Autodesk Fusion 360 part; units mm, degrees
(part 3 of 6)
  arc A18 (6.5769, 24.5337) -> (4.7192, 24.9577) centre (0, 0) ccw
  spline S7 degree 5 poles (4.7192, 24.9577) (4.7084, 24.9471) (4.6868, 24.9257) (4.6546, 24.8937) (4.6118, 24.8508) (4.5587, 24.797) (4.5059, 24.743) (4.4535, 24.6888) (4.4015, 24.6344) (4.3499, 24.5799) (4.2987, 24.5251) (4.2478, 24.4701) (4.1974, 24.415) (4.1473, 24.3596) (4.0977, 24.3041) (4.0484, 24.2484) (3.9995, 24.1925) (3.951, 24.1364) (3.903, 24.0801) (3.8553, 24.0236) (3.8081, 23.9669) (3.7613, 23.9101) (3.7149, 23.8531) (3.6689, 23.7958) (3.6234, 23.7385) (3.5783, 23.6809) (3.5336, 23.6231) (3.4894, 23.5652) (3.4456, 23.5071) (3.4023, 23.4488) (3.3594, 23.3903) (3.317, 23.3317) (3.275, 23.2729) (3.2335, 23.2139) (3.1925, 23.1547) (3.152, 23.0954) (3.1119, 23.0358) (3.0724, 22.9762) (3.0333, 22.9163) (2.9947, 22.8563) (2.9567, 22.7961) (2.9191, 22.7357) (2.8821, 22.6752) (2.8457, 22.6145) (2.8097, 22.5536) (2.7744, 22.4926) (2.7395, 22.4314) (2.7052, 22.37) (2.6715, 22.3085) (2.6383, 22.2468) (2.6058, 22.1849) (2.5738, 22.1229) (2.5426, 22.0607) (2.512, 21.9983) (2.4821, 21.9358) (2.4528, 21.873) (2.4242, 21.8102) (2.3961, 21.7472) (2.3686, 21.684) (2.3419, 21.6207) (2.316, 21.5572) (2.2911, 21.4935) (2.2673, 21.4296) (2.2446, 21.3655) (2.2228, 21.3011) (2.2018, 21.2367) (2.1812, 21.1721) (2.1613, 21.1075) (2.142, 21.0427) (2.1241, 20.9778) (2.1085, 20.9125) (2.0984, 20.8598) (2.0926, 20.82) (2.0895, 20.7934) (2.0882, 20.78) knots -1 -1 -1 -1 -1 -1 -0.98571429 -0.97142857 -0.95714286 -0.94285714 -0.92857143 -0.91428571 -0.9 -0.88571429 -0.87142857 -0.85714286 -0.84285714 -0.82857143 -0.81428571 -0.8 -0.78571429 -0.77142857 -0.75714286 -0.74285714 -0.72857143 -0.71428571 -0.7 -0.68571429 -0.67142857 -0.65714286 -0.64285714 -0.62857143 -0.61428571 -0.6 -0.58571429 -0.57142857 -0.55714286 -0.54285714 -0.52857143 -0.51428571 -0.5 -0.48571429 -0.47142857 -0.45714286 -0.44285714 -0.42857143 -0.41428571 -0.4 -0.38571429 -0.37142857 -0.35714286 -0.34285714 -0.32857143 -0.31428571 -0.3 -0.28571429 -0.27142857 -0.25714286 -0.24285714 -0.22857143 -0.21428571 -0.2 -0.18571429 -0.17142857 -0.15714286 -0.14285714 -0.12857143 -0.11428571 -0.1 -0.08571429 -0.07142857 -0.05714286 -0.04285714 -0.02857143 -0.01428571 0 0 0 0 0 0
  line L7 (2.0882, 20.78) -> (1.988, 19.788)
  arc A19 (0.376, 18.3604) -> (1.988, 19.788) centre (0.4085, 19.9475) ccw
  arc A20 (0.376, 18.3604) -> (-0.376, 18.3604) centre (0, 0) ccw
  arc A21 (-1.988, 19.788) -> (-0.376, 18.3604) centre (-0.4085, 19.9475) ccw
  line L8 (-1.988, 19.788) -> (-2.0882, 20.78)
  spline S8 degree 5 poles (-2.0882, 20.78) (-2.0895, 20.7934) (-2.0926, 20.82) (-2.0984, 20.8598) (-2.1085, 20.9125) (-2.1241, 20.9778) (-2.142, 21.0427) (-2.1613, 21.1075) (-2.1812, 21.1721) (-2.2018, 21.2367) (-2.2228, 21.3011) (-2.2446, 21.3655) (-2.2673, 21.4296) (-2.2911, 21.4935) (-2.316, 21.5572) (-2.3419, 21.6207) (-2.3686, 21.684) (-2.3961, 21.7472) (-2.4242, 21.8102) (-2.4528, 21.873) (-2.4821, 21.9358) (-2.512, 21.9983) (-2.5426, 22.0607) (-2.5738, 22.1229) (-2.6058, 22.1849) (-2.6383, 22.2468) (-2.6715, 22.3085) (-2.7052, 22.37) (-2.7395, 22.4314) (-2.7744, 22.4926) (-2.8097, 22.5536) (-2.8457, 22.6145) (-2.8821, 22.6752) (-2.9191, 22.7357) (-2.9567, 22.7961) (-2.9947, 22.8563) (-3.0333, 22.9163) (-3.0724, 22.9762) (-3.1119, 23.0358) (-3.152, 23.0954) (-3.1925, 23.1547) (-3.2335, 23.2139) (-3.275, 23.2729) (-3.317, 23.3317) (-3.3594, 23.3903) (-3.4023, 23.4488) (-3.4456, 23.5071) (-3.4894, 23.5652) (-3.5336, 23.6231) (-3.5783, 23.6809) (-3.6234, 23.7385) (-3.6689, 23.7958) (-3.7149, 23.8531) (-3.7613, 23.9101) (-3.8081, 23.9669) (-3.8553, 24.0236) (-3.903, 24.0801) (-3.951, 24.1364) (-3.9995, 24.1925) (-4.0484, 24.2484) (-4.0977, 24.3041) (-4.1473, 24.3596) (-4.1974, 24.415) (-4.2478, 24.4701) (-4.2987, 24.5251) (-4.3499, 24.5799) (-4.4015, 24.6344) (-4.4535, 24.6888) (-4.5059, 24.743) (-4.5587, 24.797) (-4.6118, 24.8508) (-4.6546, 24.8937) (-4.6868, 24.9257) (-4.7084, 24.9471) (-4.7192, 24.9577) knots 0 0 0 0 0 0 0.01428571 0.02857143 0.04285714 0.05714286 0.07142857 0.08571429 0.1 0.11428571 0.12857143 0.14285714 0.15714286 0.17142857 0.18571429 0.2 0.21428571 0.22857143 0.24285714 0.25714286 0.27142857 0.28571429 0.3 0.31428571 0.32857143 0.34285714 0.35714286 0.37142857 0.38571429 0.4 0.41428571 0.42857143 0.44285714 0.45714286 0.47142857 0.48571429 0.5 0.51428571 0.52857143 0.54285714 0.55714286 0.57142857 0.58571429 0.6 0.61428571 0.62857143 0.64285714 0.65714286 0.67142857 0.68571429 0.7 0.71428571 0.72857143 0.74285714 0.75714286 0.77142857 0.78571429 0.8 0.81428571 0.82857143 0.84285714 0.85714286 0.87142857 0.88571429 0.9 0.91428571 0.92857143 0.94285714 0.95714286 0.97142857 0.98571429 1 1 1 1 1 1
  arc A22 (-4.7192, 24.9577) -> (-6.5769, 24.5337) centre (0, 0) ccw
  spline S9 degree 5 poles (-6.5769, 24.5337) (-6.582, 24.5195) (-6.5922, 24.4909) (-6.6073, 24.448) (-6.6273, 24.3908) (-6.6518, 24.3193) (-6.6759, 24.2477) (-6.6996, 24.1762) (-6.7228, 24.1046) (-6.7457, 24.0331) (-6.768, 23.9615) (-6.79, 23.8899) (-6.8115, 23.8183) (-6.8326, 23.7467) (-6.8533, 23.6751) (-6.8735, 23.6036) (-6.8933, 23.532) (-6.9126, 23.4604) (-6.9315, 23.3888) (-6.9499, 23.3173) (-6.9679, 23.2457) (-6.9854, 23.1742) (-7.0024, 23.1027) (-7.019, 23.0312) (-7.0352, 22.9597) (-7.0508, 22.8883) (-7.066, 22.8169) (-7.0807, 22.7455) (-7.095, 22.6741) (-7.1087, 22.6028) (-7.122, 22.5315) (-7.1348, 22.4603) (-7.147, 22.3891) (-7.1588, 22.3179) (-7.1701, 22.2468) (-7.1809, 22.1758) (-7.1911, 22.1048) (-7.2009, 22.0339) (-7.2101, 21.963) (-7.2188, 21.8922) (-7.227, 21.8214) (-7.2346, 21.7507) (-7.2417, 21.6801) (-7.2482, 21.6096) (-7.2542, 21.5392) (-7.2595, 21.4689) (-7.2644, 21.3986) (-7.2687, 21.3284) (-7.2724, 21.2583) (-7.2755, 21.1884) (-7.278, 21.1185) (-7.2798, 21.0488) (-7.281, 20.9792) (-7.2814, 20.9097) (-7.2813, 20.8404) (-7.2804, 20.7712) (-7.279, 20.7021) (-7.277, 20.6332) (-7.2743, 20.5644) (-7.2709, 20.4957) (-7.2667, 20.4273) (-7.2615, 20.3591) (-7.2552, 20.2911) (-7.2478, 20.2235) (-7.2395, 20.1561) (-7.2305, 20.0889) (-7.221, 20.0218) (-7.211, 19.9549) (-7.2002, 19.8882) (-7.1881, 19.8219) (-7.1739, 19.7563) (-7.1601, 19.7045) (-7.1481, 19.6661) (-7.1393, 19.6408) (-7.1347, 19.6282) knots -1 -1 -1 -1 -1 -1 -0.98571429 -0.97142857 -0.95714286 -0.94285714 -0.92857143 -0.91428571 -0.9 -0.88571429 -0.87142857 -0.85714286 -0.84285714 -0.82857143 -0.81428571 -0.8 -0.78571429 -0.77142857 -0.75714286 -0.74285714 -0.72857143 -0.71428571 -0.7 -0.68571429 -0.67142857 -0.65714286 -0.64285714 -0.62857143 -0.61428571 -0.6 -0.58571429 -0.57142857 -0.55714286 -0.54285714 -0.52857143 -0.51428571 -0.5 -0.48571429 -0.47142857 -0.45714286 -0.44285714 -0.42857143 -0.41428571 -0.4 -0.38571429 -0.37142857 -0.35714286 -0.34285714 -0.32857143 -0.31428571 -0.3 -0.28571429 -0.27142857 -0.25714286 -0.24285714 -0.22857143 -0.21428571 -0.2 -0.18571429 -0.17142857 -0.15714286 -0.14285714 -0.12857143 -0.11428571 -0.1 -0.08571429 -0.07142857 -0.05714286 -0.04285714 -0.02857143 -0.01428571 0 0 0 0 0 0
  line L9 (-7.1347, 19.6282) -> (-6.7946, 18.6909)
  arc A23 (-7.6275, 16.7053) -> (-6.7946, 18.6909) centre (-8.2868, 18.1493) ccw
  arc A24 (-7.6275, 16.7053) -> (-8.305, 16.379) centre (0, 0) ccw
  arc A25 (-10.3768, 16.9658) -> (-8.305, 16.379) centre (-9.023, 17.7948) ccw
  line L10 (-10.3768, 16.9658) -> (-10.8975, 17.8161)
  spline S10 degree 5 poles (-10.8975, 17.8161) (-10.9045, 17.8276) (-10.9188, 17.8502) (-10.9414, 17.8836) (-10.9733, 17.9266) (-11.0157, 17.9787) (-11.06, 18.0295) (-11.1054, 18.0794) (-11.1515, 18.129) (-11.198, 18.1783) (-11.2449, 18.2272) (-11.2924, 18.2757) (-11.3407, 18.3237) (-11.3899, 18.3709) (-11.44, 18.4175) (-11.4908, 18.4635) (-11.5424, 18.5089) (-11.5946, 18.5539) (-11.6472, 18.5985) (-11.7003, 18.6427) (-11.7539, 18.6865) (-11.808, 18.7299) (-11.8626, 18.7728) (-11.9177, 18.8153) (-11.9734, 18.8573) (-12.0296, 18.8989) (-12.0862, 18.9401) (-12.1433, 18.9809) (-12.2008, 19.0213) (-12.2588, 19.0614) (-12.3171, 19.101) (-12.3759, 19.1403) (-12.4351, 19.1791) (-12.4947, 19.2176) (-12.5547, 19.2557) (-12.6151, 19.2934) (-12.6759, 19.3308) (-12.7371, 19.3678) (-12.7986, 19.4044) (-12.8605, 19.4406) (-12.9228, 19.4765) (-12.9854, 19.512) (-13.0484, 19.5472) (-13.1117, 19.5819) (-13.1754, 19.6164) (-13.2394, 19.6504) (-13.3037, 19.6842) (-13.3684, 19.7175) (-13.4334, 19.7505) (-13.4987, 19.7832) (-13.5643, 19.8155) (-13.6302, 19.8474) (-13.6965, 19.879) (-13.763, 19.9103) (-13.8298, 19.9412) (-13.897, 19.9717) (-13.9644, 20.0019) (-14.0321, 20.0318) (-14.1001, 20.0613) (-14.1684, 20.0905) (-14.237, 20.1193) (-14.3059, 20.1478) (-14.375, 20.176) (-14.4444, 20.2038) (-14.514, 20.2312) (-14.584, 20.2583) (-14.6541, 20.2851) (-14.7246, 20.3115) (-14.7953, 20.3376) (-14.8662, 20.3634) (-14.9374, 20.3888) (-14.9946, 20.4089) (-15.0376, 20.4238) (-15.0663, 20.4336) (-15.0806, 20.4385) knots 0 0 0 0 0 0 0.01428571 0.02857143 0.04285714 0.05714286 0.07142857 0.08571429 0.1 0.11428571 0.12857143 0.14285714 0.15714286 0.17142857 0.18571429 0.2 0.21428571 0.22857143 0.24285714 0.25714286 0.27142857 0.28571429 0.3 0.31428571 0.32857143 0.34285714 0.35714286 0.37142857 0.38571429 0.4 0.41428571 0.42857143 0.44285714 0.45714286 0.47142857 0.48571429 0.5 0.51428571 0.52857143 0.54285714 0.55714286 0.57142857 0.58571429 0.6 0.61428571 0.62857143 0.64285714 0.65714286 0.67142857 0.68571429 0.7 0.71428571 0.72857143 0.74285714 0.75714286 0.77142857 0.78571429 0.8 0.81428571 0.82857143 0.84285714 0.85714286 0.87142857 0.88571429 0.9 0.91428571 0.92857143 0.94285714 0.95714286 0.97142857 0.98571429 1 1 1 1 1 1
  arc A26 (-15.0806, 20.4385) -> (-16.5703, 19.2505) centre (0, 0) ccw
  spline S11 degree 5 poles (-16.5703, 19.2505) (-16.5688, 19.2354) (-16.5655, 19.2053) (-16.5606, 19.16) (-16.5537, 19.0999) (-16.5448, 19.0248) (-16.5355, 18.9499) (-16.5258, 18.8752) (-16.5157, 18.8006) (-16.5052, 18.7262) (-16.4943, 18.652) (-16.483, 18.578) (-16.4714, 18.5041) (-16.4593, 18.4305) (-16.4469, 18.357) (-16.434, 18.2838) (-16.4208, 18.2107) (-16.4071, 18.1378) (-16.3931, 18.0652) (-16.3786, 17.9927) (-16.3638, 17.9204) (-16.3485, 17.8484) (-16.3329, 17.7766) (-16.3168, 17.705) (-16.3003, 17.6336) (-16.2834, 17.5624) (-16.2661, 17.4915) (-16.2484, 17.4208) (-16.2303, 17.3503) (-16.2117, 17.2801) (-16.1927, 17.2101) (-16.1733, 17.1404) (-16.1535, 17.0709) (-16.1333, 17.0017) (-16.1126, 16.9327) (-16.0914, 16.864) (-16.0699, 16.7956) (-16.0479, 16.7275) (-16.0255, 16.6596) (-16.0026, 16.592) (-15.9792, 16.5247) (-15.9555, 16.4578) (-15.9312, 16.3911) (-15.9065, 16.3247) (-15.8813, 16.2587) (-15.8556, 16.193) (-15.8295, 16.1276) (-15.8029, 16.0625) (-15.7758, 15.9977) (-15.7483, 15.9334) (-15.7202, 15.8693) (-15.6916, 15.8057) (-15.6624, 15.7425) (-15.6327, 15.6797) (-15.6025, 15.6173) (-15.5717, 15.5553) (-15.5404, 15.4937) (-15.5087, 15.4325) (-15.4765, 15.3716) (-15.4436, 15.3113) (-15.4101, 15.2514) (-15.3758, 15.1922) (-15.3407, 15.1338) (-15.3047, 15.076) (-15.268, 15.0189) (-15.2307, 14.9622) (-15.193, 14.906) (-15.155, 14.85) (-15.1163, 14.7946) (-15.0767, 14.7401) (-15.0354, 14.6872) (-15.0005, 14.6465) (-14.973, 14.6171) (-14.9541, 14.5981) (-14.9445, 14.5887) knots -1 -1 -1 -1 -1 -1 -0.98571429 -0.97142857 -0.95714286 -0.94285714 -0.92857143 -0.91428571 -0.9 -0.88571429 -0.87142857 -0.85714286 -0.84285714 -0.82857143 -0.81428571 -0.8 -0.78571429 -0.77142857 -0.75714286 -0.74285714 -0.72857143 -0.71428571 -0.7 -0.68571429 -0.67142857 -0.65714286 -0.64285714 -0.62857143 -0.61428571 -0.6 -0.58571429 -0.57142857 -0.55714286 -0.54285714 -0.52857143 -0.51428571 -0.5 -0.48571429 -0.47142857 -0.45714286 -0.44285714 -0.42857143 -0.41428571 -0.4 -0.38571429 -0.37142857 -0.35714286 -0.34285714 -0.32857143 -0.31428571 -0.3 -0.28571429 -0.27142857 -0.25714286 -0.24285714 -0.22857143 -0.21428571 -0.2 -0.18571429 -0.17142857 -0.15714286 -0.14285714 -0.12857143 -0.11428571 -0.1 -0.08571429 -0.07142857 -0.05714286 -0.04285714 -0.02857143 -0.01428571 0 0 0 0 0 0
  line L11 (-14.9445, 14.5887) -> (-14.2314, 13.8919)
  arc A27 (-14.1203, 11.7415) -> (-14.2314, 13.8919) centre (-15.3409, 12.7565) ccw
  arc A28 (-14.1203, 11.7415) -> (-14.5891, 11.1535) centre (0, 0) ccw
  arc A29 (-16.7104, 10.7834) -> (-14.5891, 11.1535) centre (-15.8503, 12.1177) ccw
  line L12 (-16.7104, 10.7834) -> (-17.5484, 11.3235)
  spline S12 degree 5 poles (-17.5484, 11.3235) (-17.5597, 11.3308) (-17.5825, 11.345) (-17.6172, 11.3652) (-17.6646, 11.3902) (-17.7255, 11.4187) (-17.7874, 11.4452) (-17.85, 11.4706) (-17.913, 11.4952) (-17.9763, 11.5194) (-18.0398, 11.5432) (-18.1037, 11.5663) (-18.168, 11.5885) (-18.2328, 11.6097) (-18.2981, 11.63) (-18.3639, 11.6493) (-18.4301, 11.6679) (-18.4966, 11.6858) (-18.5633, 11.7031) (-18.6304, 11.7199) (-18.6976, 11.7361) (-18.7652, 11.7517) (-18.833, 11.7667) (-18.9011, 11.7811) (-18.9695, 11.7948) (-19.0382, 11.8079) (-19.1071, 11.8205) (-19.1762, 11.8324) (-19.2456, 11.8439) (-19.3152, 11.8548) (-19.385, 11.8652) (-19.455, 11.8751) (-19.5252, 11.8844) (-19.5956, 11.8932) (-19.6662, 11.9015) (-19.7369, 11.9093) (-19.8079, 11.9166) (-19.8791, 11.9233) (-19.9504, 11.9296) (-20.0219, 11.9354) (-20.0936, 11.9407) (-20.1654, 11.9455) (-20.2374, 11.9499) (-20.3095, 11.9538) (-20.3818, 11.9572) (-20.4543, 11.9601) (-20.5269, 11.9625) (-20.5996, 11.9645) (-20.6725, 11.9661) (-20.7455, 11.9672) (-20.8186, 11.9678) (-20.8919, 11.968) (-20.9653, 11.9677) (-21.0388, 11.967) (-21.1124, 11.9658) (-21.1862, 11.9642) (-21.26, 11.9622) (-21.334, 11.9597) (-21.4081, 11.9568) (-21.4823, 11.9535) (-21.5566, 11.9497) (-21.6309, 11.9455) (-21.7054, 11.9408) (-21.78, 11.9358) (-21.8547, 11.9303) (-21.9295, 11.9244) (-22.0043, 11.9181) (-22.0792, 11.9113) (-22.1543, 11.9041) (-22.2294, 11.8966) (-22.3045, 11.8886) (-22.3647, 11.8818) (-22.4099, 11.8766) (-22.4401, 11.8731) (-22.4551, 11.8712) knots 0 0 0 0 0 0 0.01428571 0.02857143 0.04285714 0.05714286 0.07142857 0.08571429 0.1 0.11428571 0.12857143 0.14285714 0.15714286 0.17142857 0.18571429 0.2 0.21428571 0.22857143 0.24285714 0.25714286 0.27142857 0.28571429 0.3 0.31428571 0.32857143 0.34285714 0.35714286 0.37142857 0.38571429 0.4 0.41428571 0.42857143 0.44285714 0.45714286 0.47142857 0.48571429 0.5 0.51428571 0.52857143 0.54285714 0.55714286 0.57142857 0.58571429 0.6 0.61428571 0.62857143 0.64285714 0.65714286 0.67142857 0.68571429 0.7 0.71428571 0.72857143 0.74285714 0.75714286 0.77142857 0.78571429 0.8 0.81428571 0.82857143 0.84285714 0.85714286 0.87142857 0.88571429 0.9 0.91428571 0.92857143 0.94285714 0.95714286 0.97142857 0.98571429 1 1 1 1 1 1
  arc A30 (-22.4551, 11.8712) -> (-23.2819, 10.1545) centre (0, 0) ccw
  spline S13 degree 5 poles (-23.2819, 10.1545) (-23.2739, 10.1416) (-23.2579, 10.1158) (-23.2338, 10.0772) (-23.2015, 10.026) (-23.1609, 9.9622) (-23.12, 9.8988) (-23.0788, 9.8357) (-23.0374, 9.7729) (-22.9956, 9.7104) (-22.9537, 9.6483) (-22.9114, 9.5865) (-22.8688, 9.525) (-22.826, 9.4639) (-22.7829, 9.4031) (-22.7396, 9.3426) (-22.6959, 9.2826) (-22.652, 9.2228) (-22.6078, 9.1634) (-22.5634, 9.1044) (-22.5186, 9.0458) (-22.4736, 8.9875) (-22.4284, 8.9296) (-22.3828, 8.872) (-22.337, 8.8148) (-22.2909, 8.7581) (-22.2445, 8.7017) (-22.1979, 8.6456) (-22.151, 8.59) (-22.1038, 8.5348) (-22.0563, 8.48) (-22.0086, 8.4256) (-21.9606, 8.3716) (-21.9123, 8.318) (-21.8638, 8.2649) (-21.8149, 8.2122) (-21.7658, 8.1599) (-21.7164, 8.108) (-21.6668, 8.0566) (-21.6168, 8.0056) (-21.5666, 7.9551) (-21.5161, 7.9051) (-21.4653, 7.8556) (-21.4143, 7.8065) (-21.3629, 7.7579) (-21.3113, 7.7099) (-21.2594, 7.6623) (-21.2072, 7.6152) (-21.1547, 7.5686) (-21.1019, 7.5225) (-21.0489, 7.477) (-20.9955, 7.4321) (-20.9418, 7.3878) (-20.8878, 7.3441) (-20.8335, 7.3011) (-20.7788, 7.2586) (-20.7239, 7.2166) (-20.6688, 7.1752) (-20.6133, 7.1344) (-20.5575, 7.0942) (-20.5014, 7.0549) (-20.4448, 7.0164) (-20.3878, 6.979) (-20.3303, 6.9426) (-20.2724, 6.907) (-20.2143, 6.8722) (-20.1559, 6.8378) (-20.0973, 6.8039) (-20.0385, 6.7707) (-19.9791, 6.7389) (-19.919, 6.7091) (-19.8699, 6.6876) (-19.8324, 6.673) (-19.8071, 6.6641) (-19.7944, 6.6598) knots -1 -1 -1 -1 -1 -1 -0.98571429 -0.97142857 -0.95714286 -0.94285714 -0.92857143 -0.91428571 -0.9 -0.88571429 -0.87142857 -0.85714286 -0.84285714 -0.82857143 -0.81428571 -0.8 -0.78571429 -0.77142857 -0.75714286 -0.74285714 -0.72857143 -0.71428571 -0.7 -0.68571429 -0.67142857 -0.65714286 -0.64285714 -0.62857143 -0.61428571 -0.6 -0.58571429 -0.57142857 -0.55714286 -0.54285714 -0.52857143 -0.51428571 -0.5 -0.48571429 -0.47142857 -0.45714286 -0.44285714 -0.42857143 -0.41428571 -0.4 -0.38571429 -0.37142857 -0.35714286 -0.34285714 -0.32857143 -0.31428571 -0.3 -0.28571429 -0.27142857 -0.25714286 -0.24285714 -0.22857143 -0.21428571 -0.2 -0.18571429 -0.17142857 -0.15714286 -0.14285714 -0.12857143 -0.11428571 -0.1 -0.08571429 -0.07142857 -0.05714286 -0.04285714 -0.02857143 -0.01428571 0 0 0 0 0 0
  line L13 (-19.7944, 6.6598) -> (-18.8495, 6.3414)
  arc A31 (-17.8163, 4.4521) -> (-18.8495, 6.3414) centre (-19.3565, 4.837) ccw
  arc A32 (-17.8163, 4.4521) -> (-17.9837, 3.719) centre (0, 0) ccw
  arc A33 (-19.7343, 2.4651) -> (-17.9837, 3.719) centre (-19.5383, 4.0405) ccw
  line L14 (-19.7343, 2.4651) -> (-20.7237, 2.5882)
  spline S14 degree 5 poles (-20.7237, 2.5882) (-20.737, 2.5898) (-20.7637, 2.5928) (-20.8037, 2.5959) (-20.8573, 2.5978) (-20.9245, 2.5971) (-20.9918, 2.5941) (-21.0592, 2.5898) (-21.1266, 2.5847) (-21.1941, 2.5791) (-21.2617, 2.5729) (-21.3292, 2.566) (-21.3968, 2.5581) (-21.4645, 2.5491) (-21.5321, 2.539) (-21.5998, 2.5279) (-21.6674, 2.5159) (-21.7351, 2.5032) (-21.8028, 2.4898) (-21.8705, 2.4759) (-21.9381, 2.4613) (-22.0057, 2.446) (-22.0734, 2.4301) (-22.141, 2.4135) (-22.2085, 2.3962) (-22.2761, 2.3782) (-22.3436, 2.3596) (-22.4111, 2.3404) (-22.4786, 2.3206) (-22.546, 2.3003) (-22.6134, 2.2794) (-22.6807, 2.2579) (-22.748, 2.2358) (-22.8153, 2.2132) (-22.8825, 2.1901) (-22.9496, 2.1664) (-23.0167, 2.1421) (-23.0838, 2.1173) (-23.1508, 2.092) (-23.2177, 2.0662) (-23.2846, 2.0399) (-23.3514, 2.0131) (-23.4181, 1.9858) (-23.4848, 1.958) (-23.5514, 1.9297) (-23.618, 1.9009) (-23.6844, 1.8716) (-23.7508, 1.8418) (-23.8171, 1.8116) (-23.8834, 1.7809) (-23.9496, 1.7498) (-24.0156, 1.7181) (-24.0817, 1.686) (-24.1476, 1.6535) (-24.2134, 1.6205) (-24.2792, 1.5871) (-24.3448, 1.5532) (-24.4104, 1.5189) (-24.4759, 1.4841) (-24.5413, 1.4489) (-24.6066, 1.4133) (-24.6718, 1.3772) (-24.7369, 1.3407) (-24.8019, 1.3038) (-24.8668, 1.2664) (-24.9316, 1.2287) (-24.9962, 1.1905) (-25.0608, 1.1519) (-25.1253, 1.1129) (-25.1897, 1.0735) (-25.2539, 1.0337) (-25.3053, 1.0015) (-25.3437, 0.9772) (-25.3693, 0.9609) (-25.3821, 0.9527) knots 0 0 0 0 0 0 0.01428571 0.02857143 0.04285714 0.05714286 0.07142857 0.08571429 0.1 0.11428571 0.12857143 0.14285714 0.15714286 0.17142857 0.18571429 0.2 0.21428571 0.22857143 0.24285714 0.25714286 0.27142857 0.28571429 0.3 0.31428571 0.32857143 0.34285714 0.35714286 0.37142857 0.38571429 0.4 0.41428571 0.42857143 0.44285714 0.45714286 0.47142857 0.48571429 0.5 0.51428571 0.52857143 0.54285714 0.55714286 0.57142857 0.58571429 0.6 0.61428571 0.62857143 0.64285714 0.65714286 0.67142857 0.68571429 0.7 0.71428571 0.72857143 0.74285714 0.75714286 0.77142857 0.78571429 0.8 0.81428571 0.82857143 0.84285714 0.85714286 0.87142857 0.88571429 0.9 0.91428571 0.92857143 0.94285714 0.95714286 0.97142857 0.98571429 1 1 1 1 1 1
  arc A34 (-25.3821, 0.9527) -> (-25.3821, -0.9527) centre (0, 0) ccw
  spline S15 degree 5 poles (-25.3821, -0.9527) (-25.3693, -0.9609) (-25.3437, -0.9772) (-25.3053, -1.0015) (-25.2539, -1.0337) (-25.1897, -1.0735) (-25.1253, -1.1129) (-25.0608, -1.1519) (-24.9962, -1.1905) (-24.9316, -1.2287) (-24.8668, -1.2664) (-24.8019, -1.3038) (-24.7369, -1.3407) (-24.6718, -1.3772) (-24.6066, -1.4133) (-24.5413, -1.4489) (-24.4759, -1.4841) (-24.4104, -1.5189) (-24.3448, -1.5532) (-24.2792, -1.5871) (-24.2134, -1.6205) (-24.1476, -1.6535) (-24.0817, -1.686) (-24.0156, -1.7181) (-23.9496, -1.7498) (-23.8834, -1.7809) (-23.8171, -1.8116) (-23.7508, -1.8418) (-23.6844, -1.8716) (-23.618, -1.9009) (-23.5514, -1.9297) (-23.4848, -1.958) (-23.4181, -1.9858) (-23.3514, -2.0131) (-23.2846, -2.0399) (-23.2177, -2.0662) (-23.1508, -2.092) (-23.0838, -2.1173) (-23.0167, -2.1421) (-22.9496, -2.1664) (-22.8825, -2.1901) (-22.8153, -2.2132) (-22.748, -2.2358) (-22.6807, -2.2579) (-22.6134, -2.2794) (-22.546, -2.3003) (-22.4786, -2.3206) (-22.4111, -2.3404) (-22.3436, -2.3596) (-22.2761, -2.3782) (-22.2085, -2.3962) (-22.141, -2.4135) (-22.0734, -2.4301) (-22.0057, -2.446) (-21.9381, -2.4613) (-21.8705, -2.4759) (-21.8028, -2.4898) (-21.7351, -2.5032) (-21.6674, -2.5159) (-21.5998, -2.5279) (-21.5321, -2.539) (-21.4645, -2.5491) (-21.3968, -2.5581) (-21.3292, -2.566) (-21.2617, -2.5729) (-21.1941, -2.5791) (-21.1266, -2.5847) (-21.0592, -2.5898) (-20.9918, -2.5941) (-20.9245, -2.5971) (-20.8573, -2.5978) (-20.8037, -2.5959) (-20.7637, -2.5928) (-20.737, -2.5898) (-20.7237, -2.5882) knots -1 -1 -1 -1 -1 -1 -0.98571429 -0.97142857 -0.95714286 -0.94285714 -0.92857143 -0.91428571 -0.9 -0.88571429 -0.87142857 -0.85714286 -0.84285714 -0.82857143 -0.81428571 -0.8 -0.78571429 -0.77142857 -0.75714286 -0.74285714 -0.72857143 -0.71428571 -0.7 -0.68571429 -0.67142857 -0.65714286 -0.64285714 -0.62857143 -0.61428571 -0.6 -0.58571429 -0.57142857 -0.55714286 -0.54285714 -0.52857143 -0.51428571 -0.5 -0.48571429 -0.47142857 -0.45714286 -0.44285714 -0.42857143 -0.41428571 -0.4 -0.38571429 -0.37142857 -0.35714286 -0.34285714 -0.32857143 -0.31428571 -0.3 -0.28571429 -0.27142857 -0.25714286 -0.24285714 -0.22857143 -0.21428571 -0.2 -0.18571429 -0.17142857 -0.15714286 -0.14285714 -0.12857143 -0.11428571 -0.1 -0.08571429 -0.07142857 -0.05714286 -0.04285714 -0.02857143 -0.01428571 0 0 0 0 0 0
  line L15 (-20.7237, -2.5882) -> (-19.7343, -2.4651)
  arc A35 (-17.9837, -3.719) -> (-19.7343, -2.4651) centre (-19.5383, -4.0405) ccw
  arc A36 (-17.9837, -3.719) -> (-17.8163, -4.4521) centre (0, 0) ccw
  arc A37 (-18.8495, -6.3414) -> (-17.8163, -4.4521) centre (-19.3565, -4.837) ccw
  line L16 (-18.8495, -6.3414) -> (-19.7944, -6.6598)
  spline S16 degree 5 poles (-19.7944, -6.6598) (-19.8071, -6.6641) (-19.8324, -6.673) (-19.8699, -6.6876) (-19.919, -6.7091) (-19.9791, -6.7389) (-20.0385, -6.7707) (-20.0973, -6.8039) (-20.1559, -6.8378) (-20.2143, -6.8722) (-20.2724, -6.907) (-20.3303, -6.9426) (-20.3878, -6.979) (-20.4448, -7.0164) (-20.5014, -7.0549) (-20.5575, -7.0942) (-20.6133, -7.1344) (-20.6688, -7.1752) (-20.7239, -7.2166) (-20.7788, -7.2586) (-20.8335, -7.3011) (-20.8878, -7.3441) (-20.9418, -7.3878) (-20.9955, -7.4321) (-21.0489, -7.477) (-21.1019, -7.5225) (-21.1547, -7.5686) (-21.2072, -7.6152) (-21.2594, -7.6623) (-21.3113, -7.7099) (-21.3629, -7.7579) (-21.4143, -7.8065) (-21.4653, -7.8556) (-21.5161, -7.9051) (-21.5666, -7.9551) (-21.6168, -8.0056) (-21.6668, -8.0566) (-21.7164, -8.108) (-21.7658, -8.1599) (-21.8149, -8.2122) (-21.8638, -8.2649) (-21.9123, -8.318) (-21.9606, -8.3716) (-22.0086, -8.4256) (-22.0563, -8.48) (-22.1038, -8.5348) (-22.151, -8.59) (-22.1979, -8.6456) (-22.2445, -8.7017) (-22.2909, -8.7581) (-22.337, -8.8148) (-22.3828, -8.872) (-22.4284, -8.9296) (-22.4736, -8.9875) (-22.5186, -9.0458) (-22.5634, -9.1044) (-22.6078, -9.1634) (-22.652, -9.2228) (-22.6959, -9.2826) (-22.7396, -9.3426) (-22.7829, -9.4031) (-22.826, -9.4639) (-22.8688, -9.525) (-22.9114, -9.5865) (-22.9537, -9.6483) (-22.9956, -9.7104) (-23.0374, -9.7729) (-23.0788, -9.8357) (-23.12, -9.8988) (-23.1609, -9.9622) (-23.2015, -10.026) (-23.2338, -10.0772) (-23.2579, -10.1158) (-23.2739, -10.1416) (-23.2819, -10.1545) knots 0 0 0 0 0 0 0.01428571 0.02857143 0.04285714 0.05714286 0.07142857 0.08571429 0.1 0.11428571 0.12857143 0.14285714 0.15714286 0.17142857 0.18571429 0.2 0.21428571 0.22857143 0.24285714 0.25714286 0.27142857 0.28571429 0.3 0.31428571 0.32857143 0.34285714 0.35714286 0.37142857 0.38571429 0.4 0.41428571 0.42857143 0.44285714 0.45714286 0.47142857 0.48571429 0.5 0.51428571 0.52857143 0.54285714 0.55714286 0.57142857 0.58571429 0.6 0.61428571 0.62857143 0.64285714 0.65714286 0.67142857 0.68571429 0.7 0.71428571 0.72857143 0.74285714 0.75714286 0.77142857 0.78571429 0.8 0.81428571 0.82857143 0.84285714 0.85714286 0.87142857 0.88571429 0.9 0.91428571 0.92857143 0.94285714 0.95714286 0.97142857 0.98571429 1 1 1 1 1 1
  arc A38 (-23.2819, -10.1545) -> (-22.4551, -11.8712) centre (0, 0) ccw
  spline S17 degree 5 poles (-22.4551, -11.8712) (-22.4401, -11.8731) (-22.4099, -11.8766) (-22.3647, -11.8818) (-22.3045, -11.8886) (-22.2294, -11.8966) (-22.1543, -11.9041) (-22.0792, -11.9113) (-22.0043, -11.9181) (-21.9295, -11.9244) (-21.8547, -11.9303) (-21.78, -11.9358) (-21.7054, -11.9408) (-21.6309, -11.9455) (-21.5566, -11.9497) (-21.4823, -11.9535) (-21.4081, -11.9568) (-21.334, -11.9597) (-21.26, -11.9622) (-21.1862, -11.9642) (-21.1124, -11.9658) (-21.0388, -11.967) (-20.9653, -11.9677) (-20.8919, -11.968) (-20.8186, -11.9678) (-20.7455, -11.9672) (-20.6725, -11.9661) (-20.5996, -11.9645) (-20.5269, -11.9625) (-20.4543, -11.9601) (-20.3818, -11.9572) (-20.3095, -11.9538) (-20.2374, -11.9499) (-20.1654, -11.9455) (-20.0936, -11.9407) (-20.0219, -11.9354) (-19.9504, -11.9296) (-19.8791, -11.9233) (-19.8079, -11.9166) (-19.7369, -11.9093) (-19.6662, -11.9015) (-19.5956, -11.8932) (-19.5252, -11.8844) (-19.455, -11.8751) (-19.385, -11.8652) (-19.3152, -11.8548) (-19.2456, -11.8439) (-19.1762, -11.8324) (-19.1071, -11.8205) (-19.0382, -11.8079) (-18.9695, -11.7948) (-18.9011, -11.7811) (-18.833, -11.7667) (-18.7652, -11.7517) (-18.6976, -11.7361) (-18.6304, -11.7199) (-18.5633, -11.7031) (-18.4966, -11.6858) (-18.4301, -11.6679) (-18.3639, -11.6493) (-18.2981, -11.63) (-18.2328, -11.6097) (-18.168, -11.5885) (-18.1037, -11.5663) (-18.0398, -11.5432) (-17.9763, -11.5194) (-17.913, -11.4952) (-17.85, -11.4706) (-17.7874, -11.4452) (-17.7255, -11.4187) (-17.6646, -11.3902) (-17.6172, -11.3652) (-17.5825, -11.345) (-17.5597, -11.3308) (-17.5484, -11.3235) knots -1 -1 -1 -1 -1 -1 -0.98571429 -0.97142857 -0.95714286 -0.94285714 -0.92857143 -0.91428571 -0.9 -0.88571429 -0.87142857 -0.85714286 -0.84285714 -0.82857143 -0.81428571 -0.8 -0.78571429 -0.77142857 -0.75714286 -0.74285714 -0.72857143 -0.71428571 -0.7 -0.68571429 -0.67142857 -0.65714286 -0.64285714 -0.62857143 -0.61428571 -0.6 -0.58571429 -0.57142857 -0.55714286 -0.54285714 -0.52857143 -0.51428571 -0.5 -0.48571429 -0.47142857 -0.45714286 -0.44285714 -0.42857143 -0.41428571 -0.4 -0.38571429 -0.37142857 -0.35714286 -0.34285714 -0.32857143 -0.31428571 -0.3 -0.28571429 -0.27142857 -0.25714286 -0.24285714 -0.22857143 -0.21428571 -0.2 -0.18571429 -0.17142857 -0.15714286 -0.14285714 -0.12857143 -0.11428571 -0.1 -0.08571429 -0.07142857 -0.05714286 -0.04285714 -0.02857143 -0.01428571 0 0 0 0 0 0
  line L17 (-17.5484, -11.3235) -> (-16.7104, -10.7834)
  arc A39 (-14.5891, -11.1535) -> (-16.7104, -10.7834) centre (-15.8503, -12.1177) ccw
  arc A40 (-14.5891, -11.1535) -> (-14.1203, -11.7415) centre (0, 0) ccw
  arc A41 (-14.2314, -13.8919) -> (-14.1203, -11.7415) centre (-15.3409, -12.7565) ccw
  line L18 (-14.2314, -13.8919) -> (-14.9445, -14.5887)
  spline S18 degree 5 poles (-14.9445, -14.5887) (-14.9541, -14.5981) (-14.973, -14.6171) (-15.0005, -14.6465) (-15.0354, -14.6872) (-15.0767, -14.7401) (-15.1163, -14.7946) (-15.155, -14.85) (-15.193, -14.906) (-15.2307, -14.9622) (-15.268, -15.0189) (-15.3047, -15.076) (-15.3407, -15.1338) (-15.3758, -15.1922) (-15.4101, -15.2514) (-15.4436, -15.3113) (-15.4765, -15.3716) (-15.5087, -15.4325) (-15.5404, -15.4937) (-15.5717, -15.5553) (-15.6025, -15.6173) (-15.6327, -15.6797) (-15.6624, -15.7425) (-15.6916, -15.8057) (-15.7202, -15.8693) (-15.7483, -15.9334) (-15.7758, -15.9977) (-15.8029, -16.0625) (-15.8295, -16.1276) (-15.8556, -16.193) (-15.8813, -16.2587) (-15.9065, -16.3247) (-15.9312, -16.3911) (-15.9555, -16.4578) (-15.9792, -16.5247) (-16.0026, -16.592) (-16.0255, -16.6596) (-16.0479, -16.7275) (-16.0699, -16.7956) (-16.0914, -16.864) (-16.1126, -16.9327) (-16.1333, -17.0017) (-16.1535, -17.0709) (-16.1733, -17.1404) (-16.1927, -17.2101) (-16.2117, -17.2801) (-16.2303, -17.3503) (-16.2484, -17.4208) (-16.2661, -17.4915) (-16.2834, -17.5624) (-16.3003, -17.6336) (-16.3168, -17.705) (-16.3329, -17.7766) (-16.3485, -17.8484) (-16.3638, -17.9204) (-16.3786, -17.9927) (-16.3931, -18.0652) (-16.4071, -18.1378) (-16.4208, -18.2107) (-16.434, -18.2838) (-16.4469, -18.357) (-16.4593, -18.4305) (-16.4714, -18.5041) (-16.483, -18.578) (-16.4943, -18.652) (-16.5052, -18.7262) (-16.5157, -18.8006) (-16.5258, -18.8752) (-16.5355, -18.9499) (-16.5448, -19.0248) (-16.5537, -19.0999) (-16.5606, -19.16) (-16.5655, -19.2053) (-16.5688, -19.2354) (-16.5703, -19.2505) knots 0 0 0 0 0 0 0.01428571 0.02857143 0.04285714 0.05714286 0.07142857 0.08571429 0.1 0.11428571 0.12857143 0.14285714 0.15714286 0.17142857 0.18571429 0.2 0.21428571 0.22857143 0.24285714 0.25714286 0.27142857 0.28571429 0.3 0.31428571 0.32857143 0.34285714 0.35714286 0.37142857 0.38571429 0.4 0.41428571 0.42857143 0.44285714 0.45714286 0.47142857 0.48571429 0.5 0.51428571 0.52857143 0.54285714 0.55714286 0.57142857 0.58571429 0.6 0.61428571 0.62857143 0.64285714 0.65714286 0.67142857 0.68571429 0.7 0.71428571 0.72857143 0.74285714 0.75714286 0.77142857 0.78571429 0.8 0.81428571 0.82857143 0.84285714 0.85714286 0.87142857 0.88571429 0.9 0.91428571 0.92857143 0.94285714 0.95714286 0.97142857 0.98571429 1 1 1 1 1 1
  arc A42 (-16.5703, -19.2505) -> (-15.0806, -20.4385) centre (0, 0) ccw
  spline S19 degree 5 poles (-15.0806, -20.4385) (-15.0663, -20.4336) (-15.0376, -20.4238) (-14.9946, -20.4089) (-14.9374, -20.3888) (-14.8662, -20.3634) (-14.7953, -20.3376) (-14.7246, -20.3115) (-14.6541, -20.2851) (-14.584, -20.2583) (-14.514, -20.2312) (-14.4444, -20.2038) (-14.375, -20.176) (-14.3059, -20.1478) (-14.237, -20.1193) (-14.1684, -20.0905) (-14.1001, -20.0613) (-14.0321, -20.0318) (-13.9644, -20.0019) (-13.897, -19.9717) (-13.8298, -19.9412) (-13.763, -19.9103) (-13.6965, -19.879) (-13.6302, -19.8474) (-13.5643, -19.8155) (-13.4987, -19.7832) (-13.4334, -19.7505) (-13.3684, -19.7175) (-13.3037, -19.6842) (-13.2394, -19.6504) (-13.1754, -19.6164) (-13.1117, -19.5819) (-13.0484, -19.5472) (-12.9854, -19.512) (-12.9228, -19.4765) (-12.8605, -19.4406) (-12.7986, -19.4044) (-12.7371, -19.3678) (-12.6759, -19.3308) (-12.6151, -19.2934) (-12.5547, -19.2557) (-12.4947, -19.2176) (-12.4351, -19.1791) (-12.3759, -19.1403) (-12.3171, -19.101) (-12.2588, -19.0614) (-12.2008, -19.0213) (-12.1433, -18.9809) (-12.0862, -18.9401) (-12.0296, -18.8989) (-11.9734, -18.8573) (-11.9177, -18.8153) (-11.8626, -18.7728) (-11.808, -18.7299) (-11.7539, -18.6865) (-11.7003, -18.6427) (-11.6472, -18.5985) (-11.5946, -18.5539) (-11.5424, -18.5089) (-11.4908, -18.4635) (-11.44, -18.4175) (-11.3899, -18.3709) (-11.3407, -18.3237) (-11.2924, -18.2757) (-11.2449, -18.2272) (-11.198, -18.1783) (-11.1515, -18.129) (-11.1054, -18.0794) (-11.06, -18.0295) (-11.0157, -17.9787) (-10.9733, -17.9266) (-10.9414, -17.8836) (-10.9188, -17.8502) (-10.9045, -17.8276) (-10.8975, -17.8161) knots -1 -1 -1 -1 -1 -1 -0.98571429 -0.97142857 -0.95714286 -0.94285714 -0.92857143 -0.91428571 -0.9 -0.88571429 -0.87142857 -0.85714286 -0.84285714 -0.82857143 -0.81428571 -0.8 -0.78571429 -0.77142857 -0.75714286 -0.74285714 -0.72857143 -0.71428571 -0.7 -0.68571429 -0.67142857 -0.65714286 -0.64285714 -0.62857143 -0.61428571 -0.6 -0.58571429 -0.57142857 -0.55714286 -0.54285714 -0.52857143 -0.51428571 -0.5 -0.48571429 -0.47142857 -0.45714286 -0.44285714 -0.42857143 -0.41428571 -0.4 -0.38571429 -0.37142857 -0.35714286 -0.34285714 -0.32857143 -0.31428571 -0.3 -0.28571429 -0.27142857 -0.25714286 -0.24285714 -0.22857143 -0.21428571 -0.2 -0.18571429 -0.17142857 -0.15714286 -0.14285714 -0.12857143 -0.11428571 -0.1 -0.08571429 -0.07142857 -0.05714286 -0.04285714 -0.02857143 -0.01428571 0 0 0 0 0 0
  line L19 (-10.8975, -17.8161) -> (-10.3768, -16.9658)
  arc A43 (-8.305, -16.379) -> (-10.3768, -16.9658) centre (-9.023, -17.7948) ccw
  arc A44 (-8.305, -16.379) -> (-7.6275, -16.7053) centre (0, 0) ccw
  arc A45 (-6.7946, -18.6909) -> (-7.6275, -16.7053) centre (-8.2868, -18.1493) ccw
  line L20 (-6.7946, -18.6909) -> (-7.1347, -19.6282)
  spline S20 degree 5 poles (-7.1347, -19.6282) (-7.1393, -19.6408) (-7.1481, -19.6661) (-7.1601, -19.7045) (-7.1739, -19.7563) (-7.1881, -19.8219) (-7.2002, -19.8882) (-7.211, -19.9549) (-7.221, -20.0218) (-7.2305, -20.0889) (-7.2395, -20.1561) (-7.2478, -20.2235) (-7.2552, -20.2911) (-7.2615, -20.3591) (-7.2667, -20.4273) (-7.2709, -20.4957) (-7.2743, -20.5644) (-7.277, -20.6332) (-7.279, -20.7021) (-7.2804, -20.7712) (-7.2813, -20.8404) (-7.2814, -20.9097) (-7.281, -20.9792) (-7.2798, -21.0488) (-7.278, -21.1185) (-7.2755, -21.1884) (-7.2724, -21.2583) (-7.2687, -21.3284) (-7.2644, -21.3986) (-7.2595, -21.4689) (-7.2542, -21.5392) (-7.2482, -21.6096) (-7.2417, -21.6801) (-7.2346, -21.7507) (-7.227, -21.8214) (-7.2188, -21.8922) (-7.2101, -21.963) (-7.2009, -22.0339) (-7.1911, -22.1048) (-7.1809, -22.1758) (-7.1701, -22.2468) (-7.1588, -22.3179) (-7.147, -22.3891) (-7.1348, -22.4603) (-7.122, -22.5315) (-7.1087, -22.6028) (-7.095, -22.6741) (-7.0807, -22.7455) (-7.066, -22.8169) (-7.0508, -22.8883) (-7.0352, -22.9597) (-7.019, -23.0312) (-7.0024, -23.1027) (-6.9854, -23.1742) (-6.9679, -23.2457) (-6.9499, -23.3173) (-6.9315, -23.3888) (-6.9126, -23.4604) (-6.8933, -23.532) (-6.8735, -23.6036) (-6.8533, -23.6751) (-6.8326, -23.7467) (-6.8115, -23.8183) (-6.79, -23.8899) (-6.768, -23.9615) (-6.7457, -24.0331) (-6.7228, -24.1046) (-6.6996, -24.1762) (-6.6759, -24.2477) (-6.6518, -24.3193) (-6.6273, -24.3908) (-6.6073, -24.448) (-6.5922, -24.4909) (-6.582, -24.5195) (-6.5769, -24.5337) knots 0 0 0 0 0 0 0.01428571 0.02857143 0.04285714 0.05714286 0.07142857 0.08571429 0.1 0.11428571 0.12857143 0.14285714 0.15714286 0.17142857 0.18571429 0.2 0.21428571 0.22857143 0.24285714 0.25714286 0.27142857 0.28571429 0.3 0.31428571 0.32857143 0.34285714 0.35714286 0.37142857 0.38571429 0.4 0.41428571 0.42857143 0.44285714 0.45714286 0.47142857 0.48571429 0.5 0.51428571 0.52857143 0.54285714 0.55714286 0.57142857 0.58571429 0.6 0.61428571 0.62857143 0.64285714 0.65714286 0.67142857 0.68571429 0.7 0.71428571 0.72857143 0.74285714 0.75714286 0.77142857 0.78571429 0.8 0.81428571 0.82857143 0.84285714 0.85714286 0.87142857 0.88571429 0.9 0.91428571 0.92857143 0.94285714 0.95714286 0.97142857 0.98571429 1 1 1 1 1 1
  arc A46 (-6.5769, -24.5337) -> (-4.7192, -24.9577) centre (0, 0) ccw
  spline S21 degree 5 poles (-4.7192, -24.9577) (-4.7084, -24.9471) (-4.6868, -24.9257) (-4.6546, -24.8937) (-4.6118, -24.8508) (-4.5587, -24.797) (-4.5059, -24.743) (-4.4535, -24.6888) (-4.4015, -24.6344) (-4.3499, -24.5799) (-4.2987, -24.5251) (-4.2478, -24.4701) (-4.1974, -24.415) (-4.1473, -24.3596) (-4.0977, -24.3041) (-4.0484, -24.2484) (-3.9995, -24.1925) (-3.951, -24.1364) (-3.903, -24.0801) (-3.8553, -24.0236) (-3.8081, -23.9669) (-3.7613, -23.9101) (-3.7149, -23.8531) (-3.6689, -23.7958) (-3.6234, -23.7385) (-3.5783, -23.6809) (-3.5336, -23.6231) (-3.4894, -23.5652) (-3.4456, -23.5071) (-3.4023, -23.4488) (-3.3594, -23.3903) (-3.317, -23.3317) (-3.275, -23.2729) (-3.2335, -23.2139) (-3.1925, -23.1547) (-3.152, -23.0954) (-3.1119, -23.0358) (-3.0724, -22.9762) (-3.0333, -22.9163) (-2.9947, -22.8563) (-2.9567, -22.7961) (-2.9191, -22.7357) (-2.8821, -22.6752) (-2.8457, -22.6145) (-2.8097, -22.5536) (-2.7744, -22.4926) (-2.7395, -22.4314) (-2.7052, -22.37) (-2.6715, -22.3085) (-2.6383, -22.2468) (-2.6058, -22.1849) (-2.5738, -22.1229) (-2.5426, -22.0607) (-2.512, -21.9983) (-2.4821, -21.9358) (-2.4528, -21.873) (-2.4242, -21.8102) (-2.3961, -21.7472) (-2.3686, -21.684) (-2.3419, -21.6207) (-2.316, -21.5572) (-2.2911, -21.4935) (-2.2673, -21.4296) (-2.2446, -21.3655) (-2.2228, -21.3011) (-2.2018, -21.2367) (-2.1812, -21.1721) (-2.1613, -21.1075) (-2.142, -21.0427) (-2.1241, -20.9778) (-2.1085, -20.9125) (-2.0984, -20.8598) (-2.0926, -20.82) (-2.0895, -20.7934) (-2.0882, -20.78) knots -1 -1 -1 -1 -1 -1 -0.98571429 -0.97142857 -0.95714286 -0.94285714 -0.92857143 -0.91428571 -0.9 -0.88571429 -0.87142857 -0.85714286 -0.84285714 -0.82857143 -0.81428571 -0.8 -0.78571429 -0.77142857 -0.75714286 -0.74285714 -0.72857143 -0.71428571 -0.7 -0.68571429 -0.67142857 -0.65714286 -0.64285714 -0.62857143 -0.61428571 -0.6 -0.58571429 -0.57142857 -0.55714286 -0.54285714 -0.52857143 -0.51428571 -0.5 -0.48571429 -0.47142857 -0.45714286 -0.44285714 -0.42857143 -0.41428571 -0.4 -0.38571429 -0.37142857 -0.35714286 -0.34285714 -0.32857143 -0.31428571 -0.3 -0.28571429 -0.27142857 -0.25714286 -0.24285714 -0.22857143 -0.21428571 -0.2 -0.18571429 -0.17142857 -0.15714286 -0.14285714 -0.12857143 -0.11428571 -0.1 -0.08571429 -0.07142857 -0.05714286 -0.04285714 -0.02857143 -0.01428571 0 0 0 0 0 0
  line L21 (-2.0882, -20.78) -> (-1.988, -19.788)
  arc A47 (-0.376, -18.3604) -> (-1.988, -19.788) centre (-0.4085, -19.9475) ccw
  arc A48 (-0.376, -18.3604) -> (0.376, -18.3604) centre (0, 0) ccw
  arc A49 (1.988, -19.788) -> (0.376, -18.3604) centre (0.4085, -19.9475) ccw
  line L22 (1.988, -19.788) -> (2.0882, -20.78)
  spline S22 degree 5 poles (2.0882, -20.78) (2.0895, -20.7934) (2.0926, -20.82) (2.0984, -20.8598) (2.1085, -20.9125) (2.1241, -20.9778) (2.142, -21.0427) (2.1613, -21.1075) (2.1812, -21.1721) (2.2018, -21.2367) (2.2228, -21.3011) (2.2446, -21.3655) (2.2673, -21.4296) (2.2911, -21.4935) (2.316, -21.5572) (2.3419, -21.6207) (2.3686, -21.684) (2.3961, -21.7472) (2.4242, -21.8102) (2.4528, -21.873) (2.4821, -21.9358) (2.512, -21.9983) (2.5426, -22.0607) (2.5738, -22.1229) (2.6058, -22.1849) (2.6383, -22.2468) (2.6715, -22.3085) (2.7052, -22.37) (2.7395, -22.4314) (2.7744, -22.4926) (2.8097, -22.5536) (2.8457, -22.6145) (2.8821, -22.6752) (2.9191, -22.7357) (2.9567, -22.7961) (2.9947, -22.8563) (3.0333, -22.9163) (3.0724, -22.9762) (3.1119, -23.0358) (3.152, -23.0954) (3.1925, -23.1547) (3.2335, -23.2139) (3.275, -23.2729) (3.317, -23.3317) (3.3594, -23.3903) (3.4023, -23.4488) (3.4456, -23.5071) (3.4894, -23.5652) (3.5336, -23.6231) (3.5783, -23.6809) (3.6234, -23.7385) (3.6689, -23.7958) (3.7149, -23.8531) (3.7613, -23.9101) (3.8081, -23.9669) (3.8553, -24.0236) (3.903, -24.0801) (3.951, -24.1364) (3.9995, -24.1925) (4.0484, -24.2484) (4.0977, -24.3041) (4.1473, -24.3596) (4.1974, -24.415) (4.2478, -24.4701) (4.2987, -24.5251) (4.3499, -24.5799) (4.4015, -24.6344) (4.4535, -24.6888) (4.5059, -24.743) (4.5587, -24.797) (4.6118, -24.8508) (4.6546, -24.8937) (4.6868, -24.9257) (4.7084, -24.9471) (4.7192, -24.9577) knots 0 0 0 0 0 0 0.01428571 0.02857143 0.04285714 0.05714286 0.07142857 0.08571429 0.1 0.11428571 0.12857143 0.14285714 0.15714286 0.17142857 0.18571429 0.2 0.21428571 0.22857143 0.24285714 0.25714286 0.27142857 0.28571429 0.3 0.31428571 0.32857143 0.34285714 0.35714286 0.37142857 0.38571429 0.4 0.41428571 0.42857143 0.44285714 0.45714286 0.47142857 0.48571429 0.5 0.51428571 0.52857143 0.54285714 0.55714286 0.57142857 0.58571429 0.6 0.61428571 0.62857143 0.64285714 0.65714286 0.67142857 0.68571429 0.7 0.71428571 0.72857143 0.74285714 0.75714286 0.77142857 0.78571429 0.8 0.81428571 0.82857143 0.84285714 0.85714286 0.87142857 0.88571429 0.9 0.91428571 0.92857143 0.94285714 0.95714286 0.97142857 0.98571429 1 1 1 1 1 1
  arc A50 (4.7192, -24.9577) -> (6.5769, -24.5337) centre (0, 0) ccw
  spline S23 degree 5 poles (6.5769, -24.5337) (6.582, -24.5195) (6.5922, -24.4909) (6.6073, -24.448) (6.6273, -24.3908) (6.6518, -24.3193) (6.6759, -24.2477) (6.6996, -24.1762) (6.7228, -24.1046) (6.7457, -24.0331) (6.768, -23.9615) (6.79, -23.8899) (6.8115, -23.8183) (6.8326, -23.7467) (6.8533, -23.6751) (6.8735, -23.6036) (6.8933, -23.532) (6.9126, -23.4604) (6.9315, -23.3888) (6.9499, -23.3173) (6.9679, -23.2457) (6.9854, -23.1742) (7.0024, -23.1027) (7.019, -23.0312) (7.0352, -22.9597) (7.0508, -22.8883) (7.066, -22.8169) (7.0807, -22.7455) (7.095, -22.6741) (7.1087, -22.6028) (7.122, -22.5315) (7.1348, -22.4603) (7.147, -22.3891) (7.1588, -22.3179) (7.1701, -22.2468) (7.1809, -22.1758) (7.1911, -22.1048) (7.2009, -22.0339) (7.2101, -21.963) (7.2188, -21.8922) (7.227, -21.8214) (7.2346, -21.7507) (7.2417, -21.6801) (7.2482, -21.6096) (7.2542, -21.5392) (7.2595, -21.4689) (7.2644, -21.3986) (7.2687, -21.3284) (7.2724, -21.2583) (7.2755, -21.1884) (7.278, -21.1185) (7.2798, -21.0488) (7.281, -20.9792) (7.2814, -20.9097) (7.2813, -20.8404) (7.2804, -20.7712) (7.279, -20.7021) (7.277, -20.6332) (7.2743, -20.5644) (7.2709, -20.4957) (7.2667, -20.4273) (7.2615, -20.3591) (7.2552, -20.2911) (7.2478, -20.2235) (7.2395, -20.1561) (7.2305, -20.0889) (7.221, -20.0218) (7.211, -19.9549) (7.2002, -19.8882) (7.1881, -19.8219) (7.1739, -19.7563) (7.1601, -19.7045) (7.1481, -19.6661) (7.1393, -19.6408) (7.1347, -19.6282) knots -1 -1 -1 -1 -1 -1 -0.98571429 -0.97142857 -0.95714286 -0.94285714 -0.92857143 -0.91428571 -0.9 -0.88571429 -0.87142857 -0.85714286 -0.84285714 -0.82857143 -0.81428571 -0.8 -0.78571429 -0.77142857 -0.75714286 -0.74285714 -0.72857143 -0.71428571 -0.7 -0.68571429 -0.67142857 -0.65714286 -0.64285714 -0.62857143 -0.61428571 -0.6 -0.58571429 -0.57142857 -0.55714286 -0.54285714 -0.52857143 -0.51428571 -0.5 -0.48571429 -0.47142857 -0.45714286 -0.44285714 -0.42857143 -0.41428571 -0.4 -0.38571429 -0.37142857 -0.35714286 -0.34285714 -0.32857143 -0.31428571 -0.3 -0.28571429 -0.27142857 -0.25714286 -0.24285714 -0.22857143 -0.21428571 -0.2 -0.18571429 -0.17142857 -0.15714286 -0.14285714 -0.12857143 -0.11428571 -0.1 -0.08571429 -0.07142857 -0.05714286 -0.04285714 -0.02857143 -0.01428571 0 0 0 0 0 0
  line L23 (7.1347, -19.6282) -> (6.7946, -18.6909)
  arc A51 (7.6275, -16.7053) -> (6.7946, -18.6909) centre (8.2868, -18.1493) ccw
  arc A52 (7.6275, -16.7053) -> (8.305, -16.379) centre (0, 0) ccw
  arc A53 (10.3768, -16.9658) -> (8.305, -16.379) centre (9.023, -17.7948) ccw
  line L24 (10.3768, -16.9658) -> (10.8975, -17.8161)
  spline S24 degree 5 poles (10.8975, -17.8161) (10.9045, -17.8276) (10.9188, -17.8502) (10.9414, -17.8836) (10.9733, -17.9266) (11.0157, -17.9787) (11.06, -18.0295) (11.1054, -18.0794) (11.1515, -18.129) (11.198, -18.1783) (11.2449, -18.2272) (11.2924, -18.2757) (11.3407, -18.3237) (11.3899, -18.3709) (11.44, -18.4175) (11.4908, -18.4635) (11.5424, -18.5089) (11.5946, -18.5539) (11.6472, -18.5985) (11.7003, -18.6427) (11.7539, -18.6865) (11.808, -18.7299) (11.8626, -18.7728) (11.9177, -18.8153) (11.9734, -18.8573) (12.0296, -18.8989) (12.0862, -18.9401) (12.1433, -18.9809) (12.2008, -19.0213) (12.2588, -19.0614) (12.3171, -19.101) (12.3759, -19.1403) (12.4351, -19.1791) (12.4947, -19.2176) (12.5547, -19.2557) (12.6151, -19.2934) (12.6759, -19.3308) (12.7371, -19.3678) (12.7986, -19.4044) (12.8605, -19.4406) (12.9228, -19.4765) (12.9854, -19.512) (13.0484, -19.5472) (13.1117, -19.5819) (13.1754, -19.6164) (13.2394, -19.6504) (13.3037, -19.6842) (13.3684, -19.7175) (13.4334, -19.7505) (13.4987, -19.7832) (13.5643, -19.8155) (13.6302, -19.8474) (13.6965, -19.879) (13.763, -19.9103) (13.8298, -19.9412) (13.897, -19.9717) (13.9644, -20.0019) (14.0321, -20.0318) (14.1001, -20.0613) (14.1684, -20.0905) (14.237, -20.1193) (14.3059, -20.1478) (14.375, -20.176) (14.4444, -20.2038) (14.514, -20.2312) (14.584, -20.2583) (14.6541, -20.2851) (14.7246, -20.3115) (14.7953, -20.3376) (14.8662, -20.3634) (14.9374, -20.3888) (14.9946, -20.4089) (15.0376, -20.4238) (15.0663, -20.4336) (15.0806, -20.4385) knots 0 0 0 0 0 0 0.01428571 0.02857143 0.04285714 0.05714286 0.07142857 0.08571429 0.1 0.11428571 0.12857143 0.14285714 0.15714286 0.17142857 0.18571429 0.2 0.21428571 0.22857143 0.24285714 0.25714286 0.27142857 0.28571429 0.3 0.31428571 0.32857143 0.34285714 0.35714286 0.37142857 0.38571429 0.4 0.41428571 0.42857143 0.44285714 0.45714286 0.47142857 0.48571429 0.5 0.51428571 0.52857143 0.54285714 0.55714286 0.57142857 0.58571429 0.6 0.61428571 0.62857143 0.64285714 0.65714286 0.67142857 0.68571429 0.7 0.71428571 0.72857143 0.74285714 0.75714286 0.77142857 0.78571429 0.8 0.81428571 0.82857143 0.84285714 0.85714286 0.87142857 0.88571429 0.9 0.91428571 0.92857143 0.94285714 0.95714286 0.97142857 0.98571429 1 1 1 1 1 1
  arc A54 (15.0806, -20.4385) -> (16.5703, -19.2505) centre (0, 0) ccw
  spline S25 degree 5 poles (16.5703, -19.2505) (16.5688, -19.2354) (16.5655, -19.2053) (16.5606, -19.16) (16.5537, -19.0999) (16.5448, -19.0248) (16.5355, -18.9499) (16.5258, -18.8752) (16.5157, -18.8006) (16.5052, -18.7262) (16.4943, -18.652) (16.483, -18.578) (16.4714, -18.5041) (16.4593, -18.4305) (16.4469, -18.357) (16.434, -18.2838) (16.4208, -18.2107) (16.4071, -18.1378) (16.3931, -18.0652) (16.3786, -17.9927) (16.3638, -17.9204) (16.3485, -17.8484) (16.3329, -17.7766) (16.3168, -17.705) (16.3003, -17.6336) (16.2834, -17.5624) (16.2661, -17.4915) (16.2484, -17.4208) (16.2303, -17.3503) (16.2117, -17.2801) (16.1927, -17.2101) (16.1733, -17.1404) (16.1535, -17.0709) (16.1333, -17.0017) (16.1126, -16.9327) (16.0914, -16.864) (16.0699, -16.7956) (16.0479, -16.7275) (16.0255, -16.6596) (16.0026, -16.592) (15.9792, -16.5247) (15.9555, -16.4578) (15.9312, -16.3911) (15.9065, -16.3247) (15.8813, -16.2587) (15.8556, -16.193) (15.8295, -16.1276) (15.8029, -16.0625) (15.7758, -15.9977) (15.7483, -15.9334) (15.7202, -15.8693) (15.6916, -15.8057) (15.6624, -15.7425) (15.6327, -15.6797) (15.6025, -15.6173) (15.5717, -15.5553) (15.5404, -15.4937) (15.5087, -15.4325) (15.4765, -15.3716) (15.4436, -15.3113) (15.4101, -15.2514) (15.3758, -15.1922) (15.3407, -15.1338) (15.3047, -15.076) (15.268, -15.0189) (15.2307, -14.9622) (15.193, -14.906) (15.155, -14.85) (15.1163, -14.7946) (15.0767, -14.7401) (15.0354, -14.6872) (15.0005, -14.6465) (14.973, -14.6171) (14.9541, -14.5981) (14.9445, -14.5887) knots -1 -1 -1 -1 -1 -1 -0.98571429 -0.97142857 -0.95714286 -0.94285714 -0.92857143 -0.91428571 -0.9 -0.88571429 -0.87142857 -0.85714286 -0.84285714 -0.82857143 -0.81428571 -0.8 -0.78571429 -0.77142857 -0.75714286 -0.74285714 -0.72857143 -0.71428571 -0.7 -0.68571429 -0.67142857 -0.65714286 -0.64285714 -0.62857143 -0.61428571 -0.6 -0.58571429 -0.57142857 -0.55714286 -0.54285714 -0.52857143 -0.51428571 -0.5 -0.48571429 -0.47142857 -0.45714286 -0.44285714 -0.42857143 -0.41428571 -0.4 -0.38571429 -0.37142857 -0.35714286 -0.34285714 -0.32857143 -0.31428571 -0.3 -0.28571429 -0.27142857 -0.25714286 -0.24285714 -0.22857143 -0.21428571 -0.2 -0.18571429 -0.17142857 -0.15714286 -0.14285714 -0.12857143 -0.11428571 -0.1 -0.08571429 -0.07142857 -0.05714286 -0.04285714 -0.02857143 -0.01428571 0 0 0 0 0 0
  line L25 (14.9445, -14.5887) -> (14.2314, -13.8919)
  arc A55 (14.1203, -11.7415) -> (14.2314, -13.8919) centre (15.3409, -12.7565) ccw
  arc A56 (14.1203, -11.7415) -> (14.5891, -11.1535) centre (0, 0) ccw
  arc A57 (16.7104, -10.7834) -> (14.5891, -11.1535) centre (15.8503, -12.1177) ccw
  line L26 (16.7104, -10.7834) -> (17.5484, -11.3235)
  spline S26 degree 5 poles (17.5484, -11.3235) (17.5597, -11.3308) (17.5825, -11.345) (17.6172, -11.3652) (17.6646, -11.3902) (17.7255, -11.4187) (17.7874, -11.4452) (17.85, -11.4706) (17.913, -11.4952) (17.9763, -11.5194) (18.0398, -11.5432) (18.1037, -11.5663) (18.168, -11.5885) (18.2328, -11.6097) (18.2981, -11.63) (18.3639, -11.6493) (18.4301, -11.6679) (18.4966, -11.6858) (18.5633, -11.7031) (18.6304, -11.7199) (18.6976, -11.7361) (18.7652, -11.7517) (18.833, -11.7667) (18.9011, -11.7811) (18.9695, -11.7948) (19.0382, -11.8079) (19.1071, -11.8205) (19.1762, -11.8324) (19.2456, -11.8439) (19.3152, -11.8548) (19.385, -11.8652) (19.455, -11.8751) (19.5252, -11.8844) (19.5956, -11.8932) (19.6662, -11.9015) (19.7369, -11.9093) (19.8079, -11.9166) (19.8791, -11.9233) (19.9504, -11.9296) (20.0219, -11.9354) (20.0936, -11.9407) (20.1654, -11.9455) (20.2374, -11.9499) (20.3095, -11.9538) (20.3818, -11.9572) (20.4543, -11.9601) (20.5269, -11.9625) (20.5996, -11.9645) (20.6725, -11.9661) (20.7455, -11.9672) (20.8186, -11.9678) (20.8919, -11.968) (20.9653, -11.9677) (21.0388, -11.967) (21.1124, -11.9658) (21.1862, -11.9642) (21.26, -11.9622) (21.334, -11.9597) (21.4081, -11.9568) (21.4823, -11.9535) (21.5566, -11.9497) (21.6309, -11.9455) (21.7054, -11.9408) (21.78, -11.9358) (21.8547, -11.9303) (21.9295, -11.9244) (22.0043, -11.9181) (22.0792, -11.9113) (22.1543, -11.9041) (22.2294, -11.8966) (22.3045, -11.8886) (22.3647, -11.8818) (22.4099, -11.8766) (22.4401, -11.8731) (22.4551, -11.8712) knots 0 0 0 0 0 0 0.01428571 0.02857143 0.04285714 0.05714286 0.07142857 0.08571429 0.1 0.11428571 0.12857143 0.14285714 0.15714286 0.17142857 0.18571429 0.2 0.21428571 0.22857143 0.24285714 0.25714286 0.27142857 0.28571429 0.3 0.31428571 0.32857143 0.34285714 0.35714286 0.37142857 0.38571429 0.4 0.41428571 0.42857143 0.44285714 0.45714286 0.47142857 0.48571429 0.5 0.51428571 0.52857143 0.54285714 0.55714286 0.57142857 0.58571429 0.6 0.61428571 0.62857143 0.64285714 0.65714286 0.67142857 0.68571429 0.7 0.71428571 0.72857143 0.74285714 0.75714286 0.77142857 0.78571429 0.8 0.81428571 0.82857143 0.84285714 0.85714286 0.87142857 0.88571429 0.9 0.91428571 0.92857143 0.94285714 0.95714286 0.97142857 0.98571429 1 1 1 1 1 1
  arc A58 (22.4551, -11.8712) -> (23.2819, -10.1545) centre (0, 0) ccw